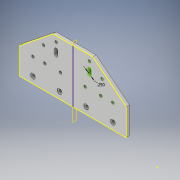
# Autodesk Inventor part: Junk Part
Saved by Autodesk Inventor 2017 (Build 210142000, 142)
## iProperties
Created: 2017-05-17
Part Number: Junk Part
Material: Generic
Document SubType Name: Modeling
Designer: User
Density: 1 g/cm^3
Appearance: Default
Author: User
Autodesk Inventor part; units mm, degrees
ref_plane "XZ Plane" through (0, 0, 0) normal (0, 1, 0) x (-1, 0, 0)
ref_plane "XY Plane" through (0, 0, 0) normal (0, 0, 1) x (1, 0, 0)
sketch "Sketch1" plane through (0, 0, 0) normal (0, 0, 1) x (1, 0, 0)
  line L0 (-262.1103, 19.715) -> (-58.9103, 19.715)
  line L1 (-58.9103, 19.715) -> (-58.9103, 70.515)
  line L2 (-58.9103, 70.515) -> (-122.4103, 121.315)
  line L3 (-122.4103, 121.315) -> (-198.6103, 121.315)
  line L4 (-198.6103, 121.315) -> (-262.1103, 70.515)
  line L5 (-262.1103, 70.515) -> (-262.1103, 19.715)
  point P0 (0, 0)
  dimension "d0" = 203.2
  dimension "d1" = 50.8
  dimension "d2" = 50.8
  dimension "d3" = 101.6
  dimension "d4" = 76.2
  dimension "d5" = 63.5
  constraints: 12 end point, 2 parallel, 1 horizontal, 1 perpendicular
  measures "d0" distance of L0.start L0.end
  measures "d1" distance of L4.end L0.start
  measures "d2" distance of L0.end L1.end
  measures "d3" distance between parallel lines of L0 L3
  measures "d4" distance of L2.end L3.end
  measures "d5" distance from line of L2.end L1
extrude "Extrusion1" add sketch "Sketch1" along normal blind 6.35
sketch "Sketch2" plane through (0, 0, 6.35) normal (0, 0, 1) x (1, 0, 0)
  line L0 (-262.1103, 19.715) -> (-58.9103, 19.715) projected
  line L1 (-58.9103, 19.715) -> (-58.9103, 70.515) projected
  line L2 (-58.9103, 70.515) -> (-122.4103, 121.315) projected
  line L3 (-122.4103, 121.315) -> (-198.6103, 121.315) projected
  line L4 (-198.6103, 121.315) -> (-262.1103, 70.515) projected
  line L5 (-262.1103, 70.515) -> (-262.1103, 19.715) projected
  point P0 (0, 0)
  point P1 (-84.3103, 32.415)
  dimension "d8" = 12.7
  dimension "d9" = 25.4
  measures "d8" distance from line of point (-84.31, 32.415) L0
  measures "d9" distance from line of point (-84.31, 32.415) L1
hole "Hole1" at (-84.3103, 32.415, 6.35) direction (0, 0, -1) diameter 4.9784 depth 19.05 tip angle 118 counterbore diameter 9.525 counterbore depth 1.27 thread size "1/4-20 UNC" class "2B" standard "ANSI Unified Screw Threads"
pattern_linear "Rectangular Pattern1" count 4 spacing 50.8 along (-1, 0, 0) of "Hole1"
sketch "Sketch3" plane through (0, 0, 6.35) normal (0, 0, 1) x (1, 0, 0)
  line L0 (-262.1103, 19.715) -> (-58.9103, 19.715) projected
  line L1 (-58.9103, 19.715) -> (-58.9103, 70.515) projected
  line L2 (-58.9103, 70.515) -> (-122.4103, 121.315) projected
  line L3 (-122.4103, 121.315) -> (-198.6103, 121.315) projected
  line L4 (-198.6103, 121.315) -> (-262.1103, 70.515) projected
  line L5 (-262.1103, 70.515) -> (-262.1103, 19.715) projected
  line L6 (-128.7603, 100.9956) -> (-128.7603, 86.3997) construction
  line L7 (-131.9353, 97.8206) -> (-131.9353, 89.5747)
  line L8 (-125.5853, 89.5747) -> (-125.5853, 97.8206)
  arc A0 (-125.5853, 97.8206) -> (-131.9353, 97.8206) centre (-128.7603, 97.8206) ccw
  arc A1 (-131.9353, 89.5747) -> (-125.5853, 89.5747) centre (-128.7603, 89.5747) ccw
  point P0 (0, 0)
  point P1 (-128.7603, 93.6976)
  point P2 (-136.9971, 64.7412)
  point P3 (-107.099, 64.7412)
  point P4 (-84.3103, 64.7412)
  point P5 (-128.7603, 110.8832)
  point P6 (-104.7448, 93.6976)
  dimension "d20" = 6.35
  constraints: 8 end point, 6 point on circle, 4 tangent, 3 point on line, 2 centre point, 1 midpoint, 1 parallel, 1 vertical
  measures "d20" diameter of A1
hole "Hole2" at (-136.9971, 64.7412, 6.35) at (-107.099, 64.7412, 6.35) at (-84.3103, 64.7412, 6.35) at (-128.7603, 110.8832, 6.35) at (-104.7448, 93.6976, 6.35) direction (0, 0, -1) diameter 4.9784 end through all thread size "1/4-20 UNC" class "2B" standard "ANSI Unified Screw Threads"
extrude "Extrusion2" cut sketch "Sketch3" against normal blind 25.4 contours A0 L8 A1 L7
sketch "Sketch4" plane through (0, 0, 6.35) normal (0, 0, 1) x (1, 0, 0)
  line L0 (-262.1103, 19.715) -> (-58.9103, 19.715) projected
  line L1 (-122.4103, 121.315) -> (-198.6103, 121.315) projected
  line L2 (-160.5103, 121.315) -> (-160.5103, 19.715)
  line L3 (-262.1103, 19.715) -> (-58.9103, 19.715) projected
  point P0 (0, 0)
  constraints: 2 end point, 2 midpoint
ref_plane "Work Plane1" through (-160.5103, 121.315, 6.35) normal (1, 0, 0) x (0, -1, 0)
mirror "Mirror1" about plane through (-160.5103, 121.315, 6.35) normal (1, 0, 0) of "Hole2", "Extrusion2"
equation "\"d2\" = d1"
equation "\"d5\" = -0.5 * d4 + 0.5 * d0"
body "Solid1"
